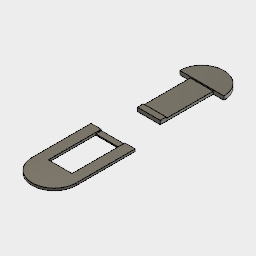
Slide (Autodesk Fusion 360 design; units mm, degrees)
Autodesk Fusion 360 part; units mm, degrees
sketch "Base" plane through (0, 0, 0) normal (0, 1, 0) x (1, 0, 0)
  line L0 (-8.4632, -15.0507) -> (6.5368, -15.0507)
  line L1 (6.5368, -15.0507) -> (6.5368, 4.9493)
  line L2 (6.5368, 4.9493) -> (-8.4632, 4.9493)
  line L3 (-8.4632, 4.9493) -> (-8.4632, -15.0507)
  arc A0 (6.5368, 4.9493) -> (-8.4632, 4.9493) centre (-0.9632, 4.9493) ccw
  arc A1 (-8.4632, -15.0507) -> (6.5368, -15.0507) centre (-0.9632, -15.0507) ccw
  line L4 (-0.9632, -15.0507) -> (-8.4632, -15.0507) construction
  line L5 (-0.9632, -15.0507) -> (6.5368, -15.0507) construction
  line L6 (-4.9632, 3) -> (3.0368, 3)
  line L7 (3.0368, 3) -> (3.0368, -13)
  line L8 (3.0368, -13) -> (-4.9632, -13)
  line L9 (-4.9632, -13) -> (-4.9632, 3)
  line L10 (-4.9632, 3) -> (3.0368, 3)
  line L11 (3.0368, 3) -> (3.0368, 4.9493)
  line L12 (3.0368, 4.9493) -> (-4.9632, 4.9493)
  line L13 (-4.9632, 4.9493) -> (-4.9632, 3)
  line L14 (-4.9632, -11) -> (3.0368, -11)
  line L15 (3.0368, -11) -> (3.0368, -13)
  line L16 (3.0368, -13) -> (-4.9632, -13)
  line L17 (-4.9632, -13) -> (-4.9632, -11)
  dimension "d2" = 15
  dimension "d3" = 20
  dimension "d4" = 180
  dimension "d17" = 8
  dimension "d18" = 3.5
  dimension "d19" = 8
  constraint horizontal L0
  constraint vertical L1
  constraint horizontal L2
  constraint vertical L3
  constraint midpoint L2 origin
  constraint midpoint L0 origin
  constraint horizontal L6
  constraint vertical L7
  constraint horizontal L8
  constraint vertical L9
  constraint horizontal L10
  constraint vertical L11
  constraint horizontal L12
  constraint vertical L13
  constraint coincident L2 origin
  constraint horizontal L14
  constraint vertical L15
  constraint horizontal L16
  constraint vertical L17
  constraint coincident L9 origin
  measures "d4" angle of L4 L5
  measures "d17" distance of L7 L9
  measures "d18" distance of L3 L9
  measures "d19" distance of L11 L13
extrude "Extrude1" add sketch "Base" along normal blind 0.8 contours L0 L1 L2 L3 L7 L8 L9 L11 L13 L15 L16 L17 | L0 A1 makes body 1
extrude "Extrude2" add sketch "Base" along normal blind 0.4 contours L2 L6 L10 L11 L12 L13 bodies 1
move_body "MoveBody1" bodies 1 to x (1, 0, 0) y (0, 1, 0) z (0, 0, 1) at (0, 0, 30)
extrude "Extrude3" add sketch "Base" along normal blind 0.8 separate body contours L2 A0 L12 | L7 L8 L9 L14 L15 L16 L17 makes body 2 at (-2.2965, 0, 11.6667) makes body 3 at (-1.7525, 0, -10.4954)
extrude "Extrude4" add sketch "Base" along normal blind 0.4 contours L2 L6 L10 L11 L12 L13 | L6 L7 L9 L10 L14 bodies 2 3
move_face "OffsetFaces1" offset -0.1 1 faces at (-4.9632, 0.4, 12.3333) on bodies 2
move_face "OffsetFaces2" offset -0.1 1 faces at (3.0368, 0.4, 12.3333) on bodies 2
sketch "Sketch3" plane through (0, 0, 0) normal (0, 1, 0) x (1, 0, 0)
sketch "Sketch4" plane through (0, 0.4, 0) normal (0, 1, 0) x (-1, 0, 0)
  line L0 (-2.9368, 11) -> (-2.9368, -4.9493)
  line L1 (-2.9368, -4.9493) -> (4.8632, -4.9493)
  line L2 (4.8632, -4.9493) -> (4.8632, 11)
  line L3 (4.8632, 11) -> (-2.9368, 11)
sketch "Sketch5" plane through (0, 0.8, 0) normal (0, 1, 0) x (-1, 0, 0)
  line L0 (-3.0368, 25.0507) -> (-3.0368, 43)
  line L1 (-3.0368, 43) -> (4.9632, 43)
  line L2 (4.9632, 43) -> (4.9632, 25.0507)
  line L3 (4.9632, 25.0507) -> (8.4632, 25.0507)
  line L4 (8.4632, 25.0507) -> (8.4632, 45.0507)
  arc A0 (8.4632, 45.0507) -> (-6.5368, 45.0507) centre (0.9632, 45.0507) ccw
  line L5 (-6.5368, 45.0507) -> (-6.5368, 25.0507)
  line L6 (-6.5368, 25.0507) -> (-3.0368, 25.0507)
  line L7 (5, 44) -> (-5, 44)
  line L8 (-5, 44) -> (-5, 50)
  line L9 (-5, 50) -> (5, 50)
  line L10 (5, 50) -> (5, 44)
  constraint horizontal L7
  constraint vertical L8
  constraint horizontal L9
  constraint vertical L10
extrude "Extrude6" add 1 faces at (-2.2632, 0, 7.0169) along direction (0, -1, 0) blind 0.5 on bodies 2 bodies 2
move_body "MoveBody2" bodies 2 to x (1, 0, 0) y (0, 1, 0) z (0, 0, 1) at (0, 0.5, 0)
